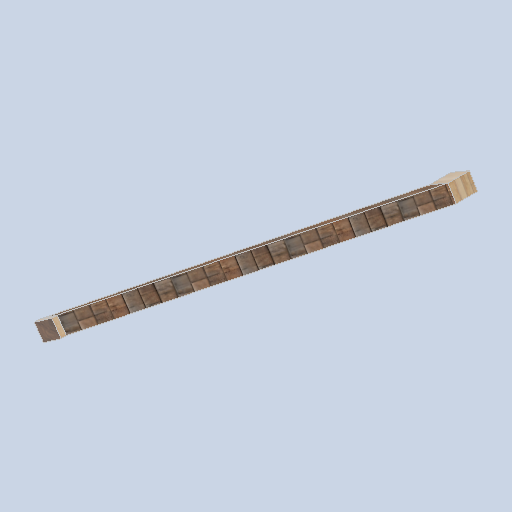
# Autodesk Inventor part: support_beam_0101
Saved by Autodesk Inventor 2024.2 (Build 282272000, 272)
## iProperties
Created: 2024-05-20
Part Number: support_beam_0101
Material: Wood (Maple)
Document SubType Name: Modeling
Designer: LOSTER_1
Density: 0.67 g/cm^3
Appearance: Natural Maple - Glossy Dark Tint
Author: LOSTER_1
Autodesk Inventor part; units mm, degrees
ref_plane "YZ Plane" through (0, 0, 0) normal (1, 0, 0) x (0, 1, 0)
ref_plane "XZ Plane" through (0, 0, 0) normal (0, 1, 0) x (-1, 0, 0)
sketch "Sketch5" plane through (0, 0, 0) normal (0, 0, 1) x (1, 0, 0)
  line L0 (801.8387, 505.4484) -> (975.0438, 605.4484)
  line L1 (975.0438, 605.4484) -> (1050.0438, 475.5446)
  line L2 (1050.0438, 475.5446) -> (876.8387, 375.5446)
  line L3 (876.8387, 375.5446) -> (801.8387, 505.4484)
  point P0 (0, 0)
  constraints: 8 end point
ref_plane "Work Plane6" through (0, 0, 3749) normal (0, 0, 1) x (1, 0, 0)
ref_plane "Work Plane5" through (0, 0, 0) normal (0, 0, 1) x (1, 0, 0)
sketch "Sketch6" plane through (0, 0, 3749) normal (0, 0, 1) x (1, 0, 0)
  line L0 (913.6134, 1349.7918) -> (1077.4438, 1464.5071) projected
  line L1 (1077.4438, 1464.5071) -> (1163.4803, 1341.6342) projected
  line L2 (999.6499, 1226.919) -> (913.6134, 1349.7918) projected
  line L3 (1163.4803, 1341.6342) -> (999.6499, 1226.919) projected
  point P0 (0, 0)
loft "Loft1" add profiles "Sketch6", "Sketch5"
sketch "Sketch7" plane through (0, 0, 0) normal (0, 0, 1) x (1, 0, 0)
  line L0 (975.0438, 605.4484) -> (1050.0438, 475.5446) projected
  line L1 (1050.0438, 475.5446) -> (876.8387, 375.5446) projected
  line L2 (801.8387, 505.4484) -> (975.0438, 605.4484) projected
  line L3 (876.8387, 375.5446) -> (801.8387, 505.4484) projected
  point P0 (0, 0)
extrude "Extrusion1" add sketch "Sketch7" against normal blind 200
sketch "Sketch8" plane through (913.6134, 1349.7918, 3749) normal (0, 0, 1) x (0.8192, 0.5736, 0)
  line L0 (0, 0) -> (200, 0) projected
  line L1 (0, -150) -> (0, 0) projected
  line L2 (200, -150) -> (0, -150) projected
  line L3 (200, 0) -> (200, -150) projected
  point P0 (-1522.5971, -581.6575)
extrude "Extrusion2" add sketch "Sketch8" along normal blind 50
body "Solid1"
